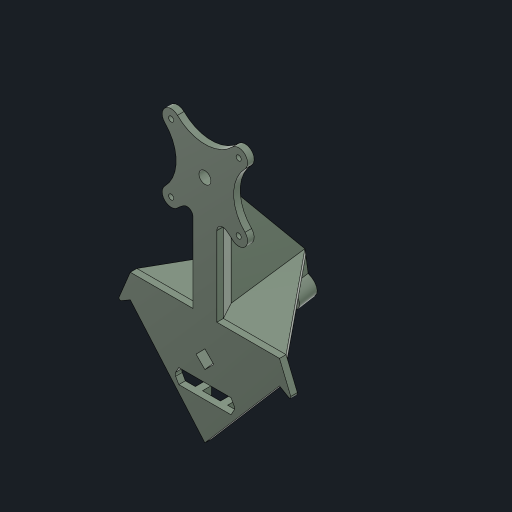
# Autodesk Inventor part: om_MotorMount_4.1
Saved by Autodesk Inventor 2023 (Build 270158000, 158)
## iProperties
Created: 2022-06-17
Part Number: om_MotorMount_4.1
Material: ABS プラスチック
Document SubType Name: Modeling
Designer: legot
Density: 1.06 g/cm^3
Appearance: 滑らか - 白
Mass: 8.05653 g
Surface Area: 73.9731 cm^2
Volume: 8.05653 cm^3
Author: legot
Autodesk Inventor part; units mm, degrees
ref_plane "YZ Plane" through (0, 0, 0) normal (1, 0, 0) x (0, 1, 0)
ref_plane "XZ Plane" through (0, 0, 0) normal (0, 1, 0) x (-1, 0, 0)
ref_plane "XY Plane" through (0, 0, 0) normal (0, 0, 1) x (1, 0, 0)
sketch "スケッチ1" plane through (0, 0, 0) normal (1, 0, 0) x (0, 1, 0)
  line L0 (40, 2.2) -> (0, 2.2)
  line L1 (0, 2.2) -> (0, 0)
  line L2 (0, 0) -> (40, 0)
  line L3 (40, 0) -> (40, 2.2)
  line L4 (0, 0) -> (25.0512, -178.2483)
  line L5 (0, 2.2) -> (-8, 2.2)
  line L6 (-8, 2.2) -> (-8, 0)
  line L7 (-8, 0) -> (0, 0)
  line L8 (25.0512, -178.2483) -> (10.1971, -180.3358)
  line L9 (-12.7472, 2.2) -> (17.6241, -179.2921)
  line L10 (-8, 2.2) -> (-37, 2.2)
  line L11 (-37, 2.2) -> (-37, 0)
  line L12 (-37, 0) -> (-8, 0)
  line L13 (-8, 0) -> (-8, 2.2)
  line L14 (40, 0) -> (4.1752, -29.708)
  line L15 (-9.3373, 0) -> (-4.1697, -30.8808)
  line L16 (4.1752, -29.708) -> (-4.1697, -30.8808)
  point P0 (-9.3373, 0)
  dimension "d0" = 2.2
  dimension "d1" = 40
  dimension "d3" = 82
  dimension "d4" = 8
  dimension "d6" = 180
  dimension "d7" = 15
  dimension "d8" = 80.5
  dimension "d11" = 30
  dimension "d24" = 3
  dimension "d78" = 37
  dimension "d102" = 58.333
  constraints: 34 end point, 5 parallel, 5 perpendicular, 3 horizontal, 3 point on line, 1 collinear, 1 midpoint
  measures "d0" distance of L2.end L0.start
  measures "d1" distance of L0.start L0.end
  measures "d3" angle of L2 L4
  measures "d4" distance of L0.end L5.end
  measures "d6" distance of L1.end L4.end
  measures "d7" distance of L4.end L8.end
  measures "d8" angle of L7 L9
  measures "d11" distance of L1.end L14.end
  measures "d24" distance between parallel lines of L15 L9
  measures "d78" distance between parallel lines of L1 L11
  measures "d102" angle of L14 L4
extrude "押し出し1" add sketch "スケッチ1" along normal blind 25 contours L1 L7 L6 L5 | L6 L12 L9 L10 | L9 L12 L11 L10
extrude "押し出し2" add sketch "スケッチ1" along normal blind 4 contours L3 L2 L1 L0
extrude "押し出し4" add sketch "スケッチ1" along normal blind 1.6 contours L14 L4 L2 | L4 L16 L15 L12 L7
sketch "スケッチ2" plane through (0, -37, 2.2) normal (0, 0, 1) x (1, 0, 0)
  line L0 (0, 0) -> (25, 0) projected
  line L1 (25, 37) -> (25, 0) projected
  line L2 (0, 0) -> (25, 29)
  point P0 (0, 37)
  point P1 (0, 29)
  constraints: 2 end point, 1 horizontal alignment, 1 point on line
extrude "押し出し5" cut sketch "スケッチ2" against normal through all
sketch "スケッチ15" plane through (4, 0, 2.2) normal (0, 0, 1) x (1, 0, 0)
  line L0 (21, 0) -> (21, -8) projected
  line L1 (21, -8) -> (24.0578, -9.7654)
  line L2 (24.77, -9.1418) -> (21, 0)
  arc A0 (24.0578, -9.7654) -> (24.77, -9.1418) centre (24.3078, -9.3324) ccw
  point P0 (-4, 0)
  point P1 (25.3301, -10.5)
  dimension "d79" = 5
  dimension "d81" = 60
  dimension "d101" = 0.5
  constraints: 4 end point, 2 point on circle, 2 point on line, 2 tangent, 1 centre point
  measures "d79" distance of L0.end point (25.33, -10.5)
  measures "d81" angle of L0 L1
  measures "d101" radius of A0
extrude "爪" add sketch "スケッチ15" against normal up to surface (2.2 mm away)
sketch "スケッチ16" plane through (4, 0, 0) normal (0, 0, -1) x (-1, 0, 0)
  line L0 (4, -37) -> (4, -9.3373) projected
  arc A0 (-5.7995, -21.4182) -> (-5.7995, -22.5818) centre (-4.75, -22) ccw
  line L1 (-4.75, -19.525) -> (-5.7995, -21.4182)
  line L2 (-4.75, -24.475) -> (-5.7995, -22.5818)
  arc A1 (-5.7995, -22.5818) -> (-5.7995, -21.4182) centre (-4.75, -22) ccw construction
  line L3 (-4.75, -19.525) -> (4, -19.525)
  line L4 (4, -19.525) -> (4, -24.475)
  line L5 (4, -24.475) -> (-4.75, -24.475)
  line L6 (-4.75, -24.475) -> (-4.75, -19.525) construction
  point P0 (4, 0)
  point P1 (4, -24.475)
  point P2 (4, -19.525)
  dimension "d84" = 15
  dimension "d85" = 8.75
  dimension "d86" = 2.4
  dimension "d97" = 4.95
  constraints: 12 end point, 4 point on circle, 2 centre point, 2 parallel, 2 tangent, 1 coincident, 1 collinear, 1 horizontal, 1 midpoint, 1 perpendicular
  measures "d84" vertical distance of L0.start A0.centre
  measures "d85" distance from line of L0 A0.centre
  measures "d86" diameter of A0
  measures "d97" distance of L2.start L1.start
extrude "押し出し17" cut sketch "スケッチ16" against normal through all
sketch "スケッチ21" plane through (1.6, 0, 0) normal (1, 0, 0) x (0, 0, -1)
  line L0 (0, -9.3373) -> (0, 40) projected
  line L1 (0, 0) -> (178.2483, 25.0512) projected
  line L2 (0, -2.0197) -> (29.9864, 2.1947)
  line L3 (29.9864, 2.1947) -> (29.708, 4.1752)
  dimension "d107" = 2
  constraints: 4 end point, 1 parallel, 1 perpendicular, 1 point on line
  measures "d107" distance between parallel lines of L1 L2
extrude "押し出し20" add sketch "スケッチ21" along normal blind 23.4
sketch "スケッチ22" plane through (1.6, 4.1752, -29.708) normal (0, 0.9902681, 0.1391731) x (1, 0, 0)
  line L0 (23.4, 0) -> (23.4, -30) projected
  line L1 (0, 0) -> (23.4, -30)
  line L2 (0, -30) -> (0, 0) projected
  line L3 (2.4, -30) -> (0, -30) projected
  line L4 (2.4, -30) -> (23.4, -30) projected
  line L5 (23.4, 0) -> (23.4, -30) projected
  line L6 (0, 0) -> (23.4, 0) projected
  point P0 (-1.6, -30)
  constraints: 2 end point
extrude "押し出し21" cut sketch "スケッチ22" against normal blind 15 contours L0 L1 L6
mirror "ミラー1" about plane through (0, -18.5, 1.1) normal (-1, 0, 0) of "押し出し1", "押し出し2", "押し出し4", "押し出し5", "爪", "押し出し17", "押し出し20", "押し出し21"
sketch "スケッチ3" plane through (4, 0, 2.2) normal (0, 0, 1) x (1, 0, 0)
  line L0 (0, 40) -> (-8, 40) projected
  circle A0 centre (-4, 40) radius 17.5 construction
  circle A1 centre (7.3137, 51.3137) radius 3
  circle A2 centre (7.3137, 28.6863) radius 3
  line L1 (7.3137, 51.3137) -> (-4, 40) construction
  line L2 (-4, 40) -> (7.3137, 28.6863) construction
  arc A3 (9.435, 49.1924) -> (9.435, 30.8076) centre (18.6274, 40) ccw
  circle A4 centre (-15.3137, 51.3137) radius 3
  arc A5 (-13.1924, 53.435) -> (5.1924, 53.435) centre (-4, 62.6274) ccw
  circle A6 centre (-15.3137, 28.6863) radius 3
  arc A7 (-17.435, 30.8076) -> (-17.435, 49.1924) centre (-26.6274, 40) ccw
  circle A8 centre (7.3137, 28.6863) radius 3
  arc A9 (5.1924, 26.565) -> (-13.1924, 26.565) centre (-4, 17.3726) ccw
  line L3 (7.3137, 28.6863) -> (18.6274, 40) construction
  point P0 (-4, 0)
  point P1 (5.1924, 26.565)
  point P2 (5.1924, 53.435)
  point P3 (-17.435, 49.1924)
  point P4 (-13.1924, 26.565)
  dimension "d123" = 6
  dimension "d25" = 35
  dimension "d124" = 16
  dimension "d127" = 360
  dimension "d129" = 45
  constraints: 8 point on circle, 6 end point, 5 centre point, 4 midpoint, 3 perpendicular, 1 coincident, 42 other
  measures "d25" diameter of A0
  measures "d124" distance of L1.start L1.end
  measures "d129" angle of L1 L0
extrude "モーター土台" add sketch "スケッチ3" against normal up to surface (2.2 mm away)
sketch "スケッチ9" plane through (4, 0, 2.2) normal (0, 0, 1) x (1, 0, 0)
  arc A0 (9.435, 49.1924) -> (5.1924, 53.435) centre (7.3137, 51.3137) ccw projected
  arc A1 (5.1924, 26.565) -> (9.435, 30.8076) centre (7.3137, 28.6863) ccw projected
  arc A2 (-13.1924, 53.435) -> (-17.435, 49.1924) centre (-15.3137, 51.3137) ccw projected
  arc A3 (-17.435, 30.8076) -> (-13.1924, 26.565) centre (-15.3137, 28.6863) ccw projected
  point P0 (-4, 0)
  constraints: 4 coincident
hole "穴1" at (11.3137, 51.3137, 2.2) at (-11.3137, 51.3137, 2.2) at (-11.3137, 28.6863, 2.2) at (11.3137, 28.6863, 2.2) direction (0, 0, -1) diameter 1.7 end through all
ref_plane "作業平面2" through (0, -12.5822, 1.2137) normal (0, 0.1650476, -0.9862856) x (-1, 0, 0)
ref_plane "作業平面1" through (0, -12.7472, 2.2) normal (0, 0.1650476, -0.9862856) x (-1, 0, 0)
sketch "スケッチ7" plane through (0, -12.5822, 1.2137) normal (0, 0.1650476, -0.9862856) x (-1, 0, 0)
  circle A0 centre (0, 0) radius 4
  point P0 (0, 12.2093)
  dimension "d38" = 8
  constraints: 1 centre point, 1 coincident
  measures "d38" diameter of A0
extrude "押し出し10" add sketch "スケッチ7" along normal blind 5
sketch "スケッチ6" plane through (0, -12.5822, 1.2137) normal (0, 0.1650476, -0.9862856) x (-1, 0, 0)
  line L0 (0, 2.9698) -> (2.9698, 0)
  line L1 (2.9698, 0) -> (0, -2.9698)
  line L2 (0, -2.9698) -> (-2.9698, 0)
  line L3 (-2.9698, 0) -> (0, 2.9698)
  point P0 (0, 12.2093)
  point P1 (0, 0)
  dimension "d35" = 4.2
  constraints: 8 end point, 2 parallel, 2 perpendicular, 2 vertical alignment, 1 horizontal alignment
  measures "d35" distance of L2.end L0.start
extrude "ロッド穴" cut sketch "スケッチ6" along normal through all both and the other way through all
sketch "スケッチ10" plane through (25, 0, 0) normal (0, 0, -1) x (-1, 0, 0)
  circle A0 centre (25, 40) radius 3
  line L0 (25, -9.7361) -> (22.0302, -12.7472) projected
  line L1 (22.0302, -12.7472) -> (25, -15.7584) projected
  line L2 (25, -15.7584) -> (27.9698, -12.7472) projected
  line L3 (27.9698, -12.7472) -> (25, -9.7361) projected
  line L4 (16.25, -24.475) -> (33.75, -24.475) projected
  line L5 (33.75, -24.475) -> (34.7995, -22.5818) projected
  arc A1 (34.7995, -22.5818) -> (34.7995, -21.4182) centre (33.75, -22) ccw projected
  line L6 (34.7995, -21.4182) -> (33.75, -19.525) projected
  line L7 (33.75, -19.525) -> (16.25, -19.525) projected
  line L8 (16.25, -19.525) -> (15.2005, -21.4182) projected
  arc A2 (15.2005, -21.4182) -> (15.2005, -22.5818) centre (16.25, -22) ccw projected
  line L9 (15.2005, -22.5818) -> (16.25, -24.475) projected
  line L10 (50, -8) -> (25, -37) projected
  line L11 (25, -37) -> (0, -8) projected
  line L12 (0, -8) -> (-3.0578, -9.7654) projected
  arc A3 (-3.77, -9.1418) -> (-3.0578, -9.7654) centre (-3.3078, -9.3324) ccw projected
  line L13 (-3.77, -9.1418) -> (0, 0) projected
  line L14 (21, 0) -> (0, 0) projected
  line L15 (21, 29.7419) -> (21, 0) projected
  line L16 (29, 29.7419) -> (29, 0) projected
  line L17 (29, 0) -> (50, 0) projected
  line L18 (53.77, -9.1418) -> (50, 0) projected
  arc A4 (53.0578, -9.7654) -> (53.77, -9.1418) centre (53.3078, -9.3324) ccw projected
  line L19 (50, -8) -> (53.0578, -9.7654) projected
  arc A5 (21, 29.7419) -> (15.8076, 26.565) centre (25, 17.3726) ccw projected
  arc A6 (11.565, 30.8076) -> (15.8076, 26.565) centre (13.6863, 28.6863) ccw projected
  arc A7 (11.565, 30.8076) -> (11.565, 49.1924) centre (2.3726, 40) ccw projected
  arc A8 (15.8076, 53.435) -> (11.565, 49.1924) centre (13.6863, 51.3137) ccw projected
  arc A9 (15.8076, 53.435) -> (34.1924, 53.435) centre (25, 62.6274) ccw projected
  arc A10 (38.435, 49.1924) -> (34.1924, 53.435) centre (36.3137, 51.3137) ccw projected
  arc A11 (38.435, 49.1924) -> (38.435, 30.8076) centre (47.6274, 40) ccw projected
  arc A12 (34.1924, 26.565) -> (38.435, 30.8076) centre (36.3137, 28.6863) ccw projected
  arc A13 (34.1924, 26.565) -> (29, 29.7419) centre (25, 17.3726) ccw projected
  point P0 (25, 0)
  dimension "d56" = 6
  constraints: 1 centre point, 1 coincident
  measures "d56" diameter of A0
extrude "押し出し12" add sketch "スケッチ10" along normal blind 3 contours A0
sketch "スケッチ11" plane through (4, 0, 2.2) normal (0, 0, 1) x (1, 0, 0)
  arc A0 (-2.4, 37.4623) -> (-5.6, 37.4623) centre (-4, 40) ccw projected
  circle A1 centre (-4, 40) radius 2
  point P0 (-4, 0)
  point P1 (-8, 40)
  point P2 (-2, 40)
  dimension "d59" = 4
  constraints: 1 centre point, 1 coincident
  measures "d59" diameter of A1
extrude "押し出し13" cut sketch "スケッチ11" against normal blind 10
ref_plane "作業平面3" through (0, -4.1697, -30.8808) normal (0, 0.1650476, -0.9862856) x (1, 0, 0)
sketch "スケッチ8" plane through (0, -4.1697, -30.8808) normal (0, 0.1650476, -0.9862856) x (1, 0, 0)
  arc A0 (1.6, -0.6661) -> (-1.6, -0.6661) centre (0, 3) ccw projected
  line L0 (2.9698, 3) -> (1.4849, 1.5151) projected
  line L1 (-1.4849, 1.5151) -> (-2.9698, 3) projected
  line L2 (0, 5.9698) -> (2.9698, 3) projected
  line L3 (-2.9698, 3) -> (0, 5.9698) projected
  line L4 (2.9698, 3) -> (0, 0.0302) projected
  line L5 (0, 0.0302) -> (-2.9698, 3) projected
  line L6 (-2.9698, 3) -> (0, 5.9698) projected
  line L7 (0, 5.9698) -> (2.9698, 3) projected
  line L8 (1.6, -0.6661) -> (1.6, 0) projected
  line L9 (1.6, 0) -> (-1.6, 0) projected
  line L10 (-1.6, 0) -> (-1.6, -0.6661) projected
  point P0 (0, -9.2093)
  point P1 (0, -9.3484)
  point P2 (2.9698, 3)
  point P3 (2.9698, 3)
  constraints: 2 other
extrude "押し出し11" add sketch "スケッチ8" against normal blind 6
fillet "フィレット2" [suppressed]
ref_plane "YZ平面" through (0, -9.653, 1.7039) normal (-1, 0, 0) x (0, 0.1650476, -0.9862856)
ref_plane "XZ平面" through (-2.9698, -12.5822, 1.2137) normal (0, -0.9862856, -0.1650476) x (0, 0.1650476, -0.9862856)
sketch "スケッチ23" plane through (0, 40, 0) normal (0, 0, -1) x (-1, 0, 0)
  line L0 (-25, -48) -> (0, -77) projected
  line L1 (8.75, -64.475) -> (-8.75, -64.475) projected
  line L2 (-8.75, -64.475) -> (-9.7995, -62.5818) projected
  arc A0 (-9.7995, -61.4182) -> (-9.7995, -62.5818) centre (-8.75, -62) ccw projected
  line L3 (-9.7995, -61.4182) -> (-8.75, -59.525) projected
  line L4 (-8.75, -59.525) -> (8.75, -59.525) projected
  line L5 (8.75, -59.525) -> (9.7995, -61.4182) projected
  arc A1 (9.7995, -62.5818) -> (9.7995, -61.4182) centre (8.75, -62) ccw projected
  line L6 (9.7995, -62.5818) -> (8.75, -64.475) projected
  line L7 (-9.5811, -58.114) -> (-11.0335, -60.7341)
  arc A2 (-11.0335, -60.7341) -> (-11.0335, -63.2659) centre (-8.75, -62) ccw
  line L8 (-11.0335, -63.2659) -> (-9.5811, -65.886)
  line L9 (-9.5811, -65.886) -> (9.5811, -65.886)
  line L10 (9.5811, -65.886) -> (11.0335, -63.2659)
  arc A3 (11.0335, -63.2659) -> (11.0335, -60.7341) centre (8.75, -62) ccw
  line L11 (11.0335, -60.7341) -> (9.5811, -58.114)
  line L12 (9.5811, -58.114) -> (-9.5811, -58.114)
  line L13 (-8.75, -59.525) -> (-9.5811, -58.114)
  line L14 (-9.5811, -65.886) -> (-8.75, -64.475)
  line L15 (9.7995, -61.4182) -> (8.75, -59.525) projected
  line L16 (9.5811, -65.886) -> (8.75, -64.475)
  line L17 (8.75, -59.525) -> (9.5811, -58.114)
  point P0 (0, -40)
  constraints: 20 end point, 4 point on circle, 2 centre point, 1 point on line, 7 other
extrude "押し出し22" [suppressed]
fillet "フィレット3" [suppressed]
fillet "フィレット4" [suppressed]
sketch "スケッチ24" plane through (8.75, -24.475, 0) normal (0, 0, -1) x (-1, 0, 0)
  line L0 (17.5, 0) -> (0, 0) projected
  line L1 (0, 0) -> (17.5, 0) projected
  line L2 (8.75, 0) -> (8.75, -12.525)
  line L3 (11.75, 0) -> (14.15, 0)
  line L4 (14.15, 0) -> (14.15, -3)
  line L5 (14.15, -3) -> (11.75, -3)
  line L6 (11.75, -3) -> (11.75, 0)
  line L7 (5.75, 0) -> (3.35, 0)
  line L8 (3.35, 0) -> (3.35, -3)
  line L9 (3.35, -3) -> (5.75, -3)
  line L10 (5.75, -3) -> (5.75, 0)
  point P0 (8.75, 24.475)
  point P1 (5.75, 0)
  point P2 (3.35, 0)
  point P3 (14.15, 0)
  point P4 (11.75, 0)
  dimension "d117" = 2.4
  dimension "d118" = 6
  dimension "d119" = 3
  constraints: 18 end point, 4 symmetric about line, 2 parallel, 2 perpendicular, 1 horizontal, 1 midpoint, 1 point on line
  measures "d117" distance of L4.end L5.end
  measures "d118" distance between parallel lines of L10 L6
  measures "d119" distance of L3.end L4.end
extrude "押し出し23" add sketch "スケッチ24" along normal blind 3
fillet "フィレット5" radius 2 2 edges at (4, 29.7419, 1.1) (-4, 29.7419, 1.1)
chamfer "面取り1" distance 5 distance2 2.4 1 edges at (-1.6, 18.7311, 0) measured on face at (-1.6, 18.7311, -0.5)
chamfer "面取り2" distance 2.4 distance2 5 1 edges at (1.6, 18.7311, 0) measured on face at (2.1, 18.7311, 0)
